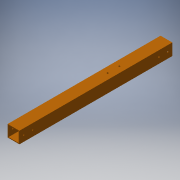
# Autodesk Inventor part: Short Side
Saved by Autodesk Inventor 2017 (Build 210142000, 142)
## iProperties
Created: 2017-01-16
Part Number: Short Side
Material: Aluminum 6061
Document SubType Name: Modeling
Designer: Ben
Density: 2.7 g/cm^3
Appearance: Orange
Mass: 137.228 g
Surface Area: 644.355 cm^2
Volume: 50.8252 cm^3
Author: Ben
Autodesk Inventor part; units mm, degrees
ref_plane "YZ Plane" through (0, 0, 0) normal (1, 0, 0) x (0, 1, 0)
ref_plane "XZ Plane" through (0, 0, 0) normal (0, 1, 0) x (-1, 0, 0)
ref_plane "XY Plane" through (0, 0, 0) normal (0, 0, 1) x (1, 0, 0)
sketch "Sketch1" plane through (0, 0, 0) normal (0, 0, 1) x (1, 0, 0)
  line L0 (0, 0) -> (-11.1125, 0) construction
  line L1 (0, 0) -> (0, 11.1125) construction
  line L2 (-11.1125, 11.1125) -> (11.1125, 11.1125)
  line L3 (11.1125, 11.1125) -> (11.1125, -11.1125)
  line L4 (11.1125, -11.1125) -> (-11.1125, -11.1125)
  line L5 (-11.1125, -11.1125) -> (-11.1125, 11.1125)
  line L6 (-12.7, 12.7) -> (12.7, 12.7)
  line L7 (12.7, 12.7) -> (12.7, -12.7)
  line L8 (12.7, -12.7) -> (-12.7, -12.7)
  line L9 (-12.7, -12.7) -> (-12.7, 12.7)
  line L10 (-11.1125, 0) -> (-12.7, 0) construction
  line L11 (0, 11.1125) -> (0, 12.7) construction
  dimension "d0" = 25.4
  dimension "d1" = 1.5875
  constraints: 24 end point, 4 horizontal, 4 midpoint, 4 parallel, 4 perpendicular, 2 vertical
  measures "d0" distance of L8.end L6.start
  measures "d1" distance of L1.end L11.end
extrude "Extrusion1" add sketch "Sketch1" along normal blind 330.2
sketch "Sketch2" plane through (12.7, -12.7, 0) normal (1, 0, 0) x (0, 0, -1)
  line L0 (0, 12.7) -> (-330.2, 12.7) construction
  line L1 (-330.2, 1.5875) -> (-330.2, 23.8125) construction
  circle A0 centre (-320.675, 12.7) radius 1.27
  circle A1 centre (-301.625, 12.7) radius 1.27
  circle A2 centre (-9.525, 12.7) radius 1.5875
  circle A3 centre (-28.575, 12.7) radius 1.5875
  dimension "d4" = 2.54
  dimension "d5" = 19.05
  dimension "d6" = 9.525
  dimension "d7" = 3.175
  dimension "d8" = 19.05
  dimension "d9" = 9.525
  constraints: 4 centre point, 4 point on line, 2 end point, 2 equal radius, 1 midpoint
  measures "d4" diameter of A0
  measures "d5" distance of A0.centre A1.centre
  measures "d6" distance from line of L1 A0.centre
  measures "d7" diameter of A2
  measures "d8" distance of A3.centre A2.centre
  measures "d9" distance of L0.start A2.centre
extrude "Extrusion2" cut sketch "Sketch2" against normal through all
sketch "Sketch3" plane through (-12.7, -12.7, 0) normal (0, -1, 0) x (1, 0, 0)
  circle A0 centre (12.7, 127) radius 1.5875
  circle A1 centre (12.7, 101.6) radius 1.5875
  line L0 (0, 0) -> (25.4, 0) construction
  line L1 (12.7, 0) -> (12.7, 101.6) construction
  line L2 (12.7, 101.6) -> (12.7, 127) construction
  line L3 (12.7, 114.3) -> (0, 114.3) construction
  line L4 (1.5875, 0) -> (1.5875, 330.2) construction
  dimension "d12" = 3.175
  dimension "d13" = 114.3
  dimension "d14" = 25.4
  constraints: 6 end point, 2 centre point, 2 perpendicular, 1 collinear, 1 equal radius, 1 midpoint
  measures "d12" diameter of A0
  measures "d13" distance between parallel lines of L0 L3
  measures "d14" distance of L1.end L2.end
extrude "Extrusion3" cut sketch "Sketch3" against normal through all
body "Solid1"
